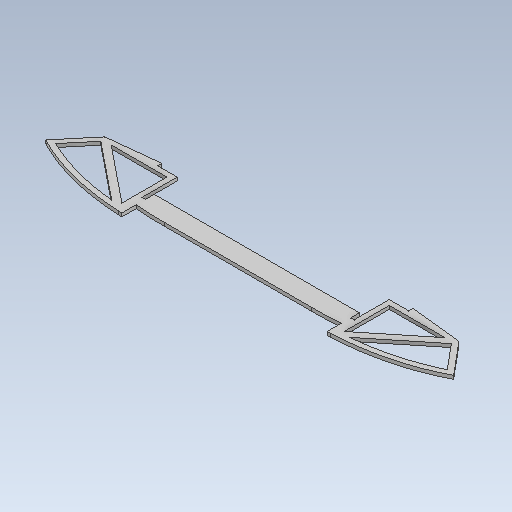
# Autodesk Inventor part: bulkhead_front
Saved by Autodesk Inventor 2020.3 (Build 243373000, 373)
## iProperties
Created: 2020-05-22
Part Number: bulkhead_front
Material: Generic
Document SubType Name: Modeling
Designer: kardo
Density: 1 g/cm^3
Appearance: Default
Mass: 5.03512 g
Surface Area: 68.3965 cm^2
Volume: 5.03512 cm^3
Author: kardo
Autodesk Inventor part; units mm, degrees
ref_plane "YZ Plane" through (0, 0, 0) normal (1, 0, 0) x (0, 1, 0)
ref_plane "XZ Plane" through (0, 0, 0) normal (0, 1, 0) x (-1, 0, 0)
ref_plane "XY Plane" through (0, 0, 0) normal (0, 0, 1) x (1, 0, 0)
derived "base_sketch.ipt"
sketch "bulkhead_front" plane through (0, 112.2, 33.6972) normal (0, 1, 0) x (-1, 0, 0)
  line L0 (-41.7231, -25.0726) -> (-11.5056, -28.3381)
  line L1 (-11.5056, -28.3381) -> (-11.5056, -25.8514)
  line L2 (-11.5056, -25.8514) -> (0, -25.8514)
  line L3 (19.176, 13.1208) -> (62.322, 13.1208)
  line L4 (-11.5056, -36.1839) -> (-34.5168, -33.6972)
  line L5 (-11.5056, -33.6972) -> (-11.5056, -36.1839)
  line L6 (0, -33.6972) -> (-11.5056, -33.6972)
  line L7 (-34.5168, -33.6972) -> (-57.528, -6.1572)
  line L8 (0, -13.7621) -> (28.764, -13.7621)
  line L9 (28.764, -20.1682) -> (62.322, -20.1682)
  line L10 (28.764, -13.7621) -> (28.764, -20.1682)
  line L11 (62.322, 13.1208) -> (62.322, -20.1682)
  line L12 (0, -13.7621) -> (0, -33.6972)
  line L13 (0, -25.8514) -> (0, -10.3406)
  line L14 (0, -10.3406) -> (62.322, -10.3406)
  line L15 (19.176, 0.918) -> (62.322, 0.918)
  line L16 (-38.352, 1.8276) -> (-38.352, 3.0228) construction
  line L17 (-19.176, 6.5076) -> (-19.176, 8.898) construction
  line L18 (0, 8.6171) -> (0, 12.2028) construction
  line L19 (-41.7231, -25.0726) -> (-57.528, -6.1572)
  line L20 (0, 8.6171) -> (0, 0)
  spline S0 degree 4 poles (-57.528, -6.1572) (-46.0483, 0.508) (-30.6129, 6.8309) (-11.2214, 11.3442) (8.3201, 13.1208) (15.5662, 13.1208) (19.176, 13.1208) knots 0 0 0 0 0 0.630279 0.815816 1 1 1 1 1
  spline S1 degree 3 poles (-57.528, -6.1572) (-39.0789, 3.4175) (-19.5173, 7.5799) (0, 8.6171) knots 0 0 0 0 1 1 1 1
  spline S2 degree 3 poles (0, 0) (6.37, 0.918) (12.773, 0.918) (19.176, 0.918) knots 0 0 0 0 1 1 1 1
  line L21 (0, 2.0028) -> (-57.528, -6.1572) construction
  point P0 (-49.746, -5.8104)
ref_plane "bulkhead_front_plane" through (0, 112.2, 33.6972) normal (0, 1, 0) x (-1, 0, 0)
sketch "Sketch2" plane through (0, 112.2, 33.6972) normal (0, 1, 0) x (-1, 0, 0)
  spline S0 degree 3 poles (-57.528, -6.1572) (-39.0789, 3.4175) (-19.5173, 7.5799) (0, 8.6171) knots 0 0 0 0 1 1 1 1 projected
  line L0 (-41.7231, -25.0726) -> (-57.528, -6.1572) projected
  line L1 (-41.7231, -25.0726) -> (-11.5056, -28.3381) projected
  line L2 (-11.5056, -25.8514) -> (0, -25.8514) projected
  line L3 (-11.5056, -28.3381) -> (-11.5056, -25.8514) projected
  line L4 (0, -25.8514) -> (0, -10.3406) projected
  line L5 (0, -10.3406) -> (62.322, -10.3406) projected
  spline S1 degree 3 poles (0, 0) (6.37, 0.918) (12.773, 0.918) (19.176, 0.918) knots 0 0 0 0 1 1 1 1 projected
  line L6 (19.176, 0.918) -> (62.322, 0.918) projected
  line L7 (0, 8.6171) -> (0, 0) projected
  line L8 (62.322, 13.1208) -> (62.322, -20.1682) projected
  line L9 (-52.7924, -7.1459) -> (-40.6712, -21.6527)
  line L10 (-41.7231, -25.0726) -> (0, 8.6171) construction
  line L11 (-3, 3.6241) -> (-3, -22.8514)
  line L12 (-3, -22.8514) -> (-35.7886, -22.8514)
  line L13 (-35.7886, -22.8514) -> (-3, 3.6241)
  line L14 (-40.6712, -21.6527) -> (-7.6212, 5.0339)
  spline S2 degree 2 poles (-52.7924, -7.1459) (-31.2795, 2.9222) (-7.6212, 5.0339) knots 0 0 0 1 1 1
  line L15 (-52.7924, -7.1459) -> (-54.0899, -4.441) construction
  line L16 (-30.7432, 0.9331) -> (-31.5102, 3.8334) construction
  line L17 (-7.6212, 5.0339) -> (-7.9157, 8.0194) construction
  line L18 (-52.7924, -7.1459) -> (-30.7432, 0.9331) construction
  line L19 (-7.6212, 5.0339) -> (-30.7432, 0.9331) construction
  line L20 (0, 8.6171) -> (2, 8.6171)
  line L21 (2, 8.6171) -> (2, 0.259)
  line L22 (0, -10.3406) -> (0, -5.1703)
  line L23 (0, -5.1703) -> (2, -5.1703)
  line L24 (2, -5.1703) -> (2, -10.3406)
  line L25 (0, -5.1703) -> (0, 0) construction
  point P0 (0, -33.6972)
  point P1 (-57.528, -9.9929)
  point P2 (-49.746, -5.8104)
  dimension "d1" = 3
  dimension "d2" = 3
  dimension "d3" = 3
  dimension "d4" = 4
  dimension "d5" = 3
  dimension "d6" = 2
  constraints: 34 end point, 4 equal length, 3 parallel, 3 vertical, 2 perpendicular, 1 collinear, 1 horizontal, 1 point on line, 13 other
  measures "d1" distance between parallel lines of L2 L12
  measures "d2" distance between parallel lines of L4 L11
  measures "d3" distance of L9.start L15.end
  measures "d4" distance between parallel lines of L13 L14
  measures "d6" distance between parallel lines of L24 L22
extrude "Extrusion1" add sketch "Sketch2" along normal blind 2 contours S0 L7 S1 L6 L8 L5 L24 L23 L22 L4 L2 L3 L1 L0 | L20 L21 S1 L7
mirror "Mirror1" about plane through (-62.322, 112.2, 23.3566) normal (-1, 0, 0) of "Extrusion1"
equation "\"d6\" = stringer_thickness"
equation "\"d7\" = bulkhead_thickness"
equation "\"stringer_thickness\" = 2"
equation "\"bulkhead_thickness\" = 2"
body "Solid1"
